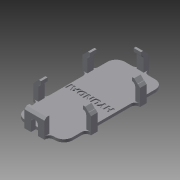
# Autodesk Inventor part: rev2
Saved by Autodesk Inventor 2015 SP2 (Build 190223200, 223)
## iProperties
Created: 2015-11-04
Part Number: rev2
Material: Generic
Document SubType Name: Modeling
Designer: KC-019
Density: 1 g/cm^3
Appearance: Default
Author: KC-019
Autodesk Inventor part; units mm, degrees
ref_plane "YZ Plane" through (0, 0, 0) normal (1, 0, 0) x (0, 1, 0)
ref_plane "XZ Plane" through (0, 0, 0) normal (0, 1, 0) x (-1, 0, 0)
ref_plane "XY Plane" through (0, 0, 0) normal (0, 0, 1) x (1, 0, 0)
sketch "Sketch1" plane through (0, 0, 0) normal (0, 0, 1) x (1, 0, 0)
  line L0 (0, 0) -> (44, 0)
  line L1 (44, 0) -> (44, 92)
  line L2 (44, 92) -> (0, 92)
  line L3 (0, 92) -> (0, 0)
  dimension "d0" = 44
  dimension "d1" = 92
  constraints: 8 end point, 2 parallel, 1 horizontal, 1 perpendicular
  measures "d0" distance of L2.end L1.end
  measures "d1" distance of L1.end L0.end
extrude "Extrusion1" add sketch "Sketch1" along normal blind 2.5
sketch "Sketch2" plane through (44, 0, 0) normal (1, 0, 0) x (0, 0, -1)
  line L0 (0, 0) -> (0, 92) projected
  line L1 (0, 46) -> (0, 23.5)
  line L2 (0, 92) -> (0, 0) projected
  line L3 (0, 46) -> (0, 68.5)
  line L4 (0, 68.5) -> (0, 65.5)
  line L5 (0, 65.5) -> (0, 71.5)
  line L6 (0, 65.5) -> (-17.1, 65.5)
  line L7 (-17.1, 65.5) -> (-17.1, 71.5)
  line L8 (-17.1, 71.5) -> (0, 71.5)
  line L9 (0, 71.5) -> (0, 65.5)
  line L10 (0, 46) -> (0, 49)
  line L11 (0, 23.5) -> (0, 20.5)
  line L12 (0, 20.5) -> (0, 26.5)
  line L13 (0, 20.5) -> (-17.1, 20.5)
  line L14 (-17.1, 20.5) -> (-17.1, 26.5)
  line L15 (-17.1, 26.5) -> (0, 26.5)
  line L16 (0, 26.5) -> (0, 20.5)
  dimension "d4" = 22.5
  dimension "d5" = 22.5
  dimension "d6" = 3
  dimension "d7" = 6
  dimension "d8" = 17.1
  dimension "d10" = 3
  dimension "d11" = 6
  dimension "d12" = 17.1
  constraints: 30 end point, 7 point on line, 4 parallel, 2 horizontal, 2 perpendicular, 1 midpoint
  measures "d4" distance of L1.start L1.end
  measures "d5" distance of L1.start L3.end
  measures "d6" distance of L3.end L4.end
  measures "d7" distance of L4.end L5.end
  measures "d8" distance of L7.end L8.end
  measures "d10" distance of L1.end L11.end
  measures "d11" distance of L11.end L12.end
  measures "d12" distance of L14.end L15.end
extrude "Extrusion2" add sketch "Sketch2" along normal blind 4.445
fillet "Fillet1" radius 4 4 edges at (44, 20.5, 1.25) (44, 65.5, 1.25) (44, 26.5, 1.25) (44, 71.5, 1.25)
chamfer "Chamfer1" distance 2 angle 45 2 edges at (48.445, 68.5, 17.1) (48.445, 23.5, 17.1)
sketch "Sketch3" plane through (0, 0, 0) normal (-1, 0, 0) x (0, 0, 1)
  line L0 (0, 92) -> (0, 0) projected
  line L1 (0, 46) -> (0, 26.5)
  line L2 (0, 46) -> (0, 65.5)
  line L3 (0, 26.5) -> (17.1, 26.5)
  line L4 (17.1, 26.5) -> (17.1, 20.5)
  line L5 (17.1, 20.5) -> (0, 20.5)
  line L6 (0, 20.5) -> (0, 26.5)
  line L7 (0, 65.5) -> (17.1, 65.5)
  line L8 (17.1, 65.5) -> (17.1, 71.5)
  line L9 (17.1, 71.5) -> (0, 71.5)
  line L10 (0, 71.5) -> (0, 65.5)
  constraints: 20 end point, 4 parallel, 2 horizontal, 2 perpendicular, 1 collinear, 1 midpoint, 1 vertical
extrude "Extrusion3" add sketch "Sketch3" along normal blind 4.445
chamfer "Chamfer2" distance 2 angle 45 2 edges at (-4.445, 68.5, 17.1) (-4.445, 23.5, 17.1)
fillet "Fillet2" radius 4 4 edges at (0, 65.5, 1.25) (0, 20.5, 1.25) (0, 71.5, 1.25) (0, 26.5, 1.25)
sketch "Sketch4" plane through (0, 92, 0) normal (0, 1, 0) x (1, 0, 0)
  line L0 (44, 0) -> (0, 0) projected
  line L1 (22, 0) -> (18.75, 0)
  line L2 (18.75, 0) -> (25.35, 0)
  line L3 (25.35, 0) -> (18.75, 0)
  line L4 (18.75, 0) -> (18.75, -17.1)
  line L5 (18.75, -17.1) -> (25.35, -17.1)
  line L6 (25.35, -17.1) -> (25.35, 0)
  dimension "d25" = 3.25
  dimension "d26" = 6.6
  dimension "d27" = 17.1
  constraints: 12 end point, 2 parallel, 2 point on line, 1 horizontal, 1 midpoint, 1 perpendicular
  measures "d25" distance of L1.start L1.end
  measures "d26" distance of L1.end L2.end
  measures "d27" distance of L4.end L3.end
extrude "Extrusion4" add sketch "Sketch4" along normal blind 4.445
fillet "Fillet3" radius 4 2 edges at (18.75, 92, 1.25) (25.35, 92, 1.25)
chamfer "Chamfer3" distance 2 angle 45 1 edges at (22.05, 96.445, 17.1)
sketch "Sketch5" plane through (0, 0, 0) normal (0, -1, 0) x (1, 0, 0)
  line L0 (25.35, 0) -> (18.75, 0) projected
  line L1 (22.05, 0) -> (24.59, 0)
  line L2 (24.59, 0) -> (18.24, 0)
  line L3 (24.59, 0) -> (30.59, 0)
  line L4 (30.59, 0) -> (30.59, 17.1)
  line L5 (30.59, 17.1) -> (24.59, 17.1)
  line L6 (24.59, 8.6399) -> (24.59, 0)
  line L7 (18.24, 0) -> (12.24, 0)
  line L8 (12.24, 0) -> (12.24, 17.1)
  line L9 (12.24, 17.1) -> (18.24, 17.1)
  line L10 (18.24, 8.6399) -> (18.24, 0)
  line L11 (24.59, 17.1) -> (18.24, 17.1)
  line L12 (21.59, 11.6399) -> (21.24, 11.6399)
  arc A0 (24.59, 8.6399) -> (21.59, 11.6399) centre (21.59, 8.6399) ccw
  arc A1 (21.24, 11.6399) -> (18.24, 8.6399) centre (21.24, 8.6399) ccw
  point P0 (0, 0)
  dimension "d34" = 2.54
  dimension "d35" = 6.35
  dimension "d36" = 6
  dimension "d37" = 17.1
  dimension "d38" = 6
  dimension "d39" = 3
  constraints: 24 end point, 5 point on line, 4 parallel, 4 point on circle, 4 tangent, 3 horizontal, 3 perpendicular, 2 centre point, 1 equal radius, 1 midpoint
  measures "d34" distance of L1.start L1.end
  measures "d35" distance of L1.end L2.end
  measures "d36" distance of L5.end L4.end
  measures "d37" distance of L4.end L3.end
  measures "d38" distance of L8.end L9.end
  measures "d39" radius of A0
extrude "Extrusion5" add sketch "Sketch5" along normal blind 4.445 contours L0 L6 A0 L12 A1 L10 L7 L8 L9 L11 L5 L4 L3
chamfer "Chamfer4" distance 2 angle 45 1 edges at (21.415, -4.445, 17.1)
fillet "Fillet4" radius 4 2 edges at (12.24, 0, 1.25) (30.59, 0, 1.25)
sketch "Sketch6" plane through (0, 0, 2.5) normal (0, 0, 1) x (1, 0, 0)
  line L0 (38.1695, 44.3728) -> (3.8106, 44.3728) construction
  line L1 (3.8106, 44.3728) -> (3.8106, 53.6459) construction
  line L2 (3.8106, 53.6459) -> (38.1695, 53.6459) construction
  line L3 (38.1695, 53.6459) -> (38.1695, 44.3728) construction
  line L4 (41.156, 49.8958) -> (40.9991, 47.6949)
  line L5 (40.9991, 47.6949) -> (40.9299, 46.0938)
  line L6 (40.9299, 46.0938) -> (40.9068, 45.3786)
  spline S0 degree 2 poles (40.9068, 45.3786) (40.9022, 45.0695) (40.9022, 44.7834) knots 0 0 0 1 1 1
  line L7 (40.9022, 44.7834) -> (40.9022, 44.3958)
  spline S1 degree 2 poles (40.9022, 44.3958) (40.2701, 44.4051) (39.9563, 44.4051) knots 0 0 0 1 1 1
  spline S2 degree 2 poles (39.9563, 44.4051) (39.7117, 44.4051) (39.1027, 44.3958) knots 0 0 0 1 1 1
  spline S3 degree 2 poles (39.1027, 44.3958) (39.1996, 45.554) (39.2273, 46.4399) knots 0 0 0 1 1 1
  line L8 (39.2273, 46.4399) -> (37.0402, 46.4399)
  spline S4 degree 2 poles (37.0402, 46.4399) (37.0217, 46.1077) (36.9848, 44.9818) (36.9848, 44.7742) knots 0 0 0 1 2 2 2
  spline S5 degree 2 poles (36.9848, 44.7742) (36.9848, 44.6681) (36.9894, 44.3958) knots 0 0 0 1 1 1
  line L9 (36.9894, 44.3958) -> (36.0343, 44.4051)
  spline S6 degree 2 poles (36.0343, 44.4051) (35.8821, 44.4051) (35.1853, 44.3958) knots 0 0 0 1 1 1
  spline S7 degree 2 poles (35.1853, 44.3958) (35.333, 46.4676) (35.416, 48.4839) (35.416, 49.8958) knots 0 0 0 1 2 2 2
  line L10 (35.416, 49.8958) -> (36.2927, 49.8866)
  spline S8 degree 2 poles (36.2927, 49.8866) (36.4911, 49.8866) (37.234, 49.8958) knots 0 0 0 1 1 1
  spline S9 degree 2 poles (37.234, 49.8958) (37.1325, 48.9361) (37.0956, 47.6626) knots 0 0 0 1 1 1
  line L11 (37.0956, 47.6626) -> (39.2919, 47.6626)
  line L12 (39.2919, 47.6626) -> (39.3611, 49.8958)
  line L13 (39.3611, 49.8958) -> (40.2931, 49.8866)
  spline S10 degree 2 poles (40.2931, 49.8866) (40.4731, 49.8866) (41.156, 49.8958) knots 0 0 0 1 1 1
  spline S11 degree 2 poles (33.2566, 49.8958) (33.2151, 49.5682) (33.1044, 48.0087) (33.1044, 47.6857) knots 0 0 0 1 2 2 2
  line L14 (33.1044, 47.6857) -> (34.9454, 44.3958)
  spline S12 degree 2 poles (34.9454, 44.3958) (34.3409, 44.4051) (33.9441, 44.4051) knots 0 0 0 1 1 1
  spline S13 degree 2 poles (33.9441, 44.4051) (33.5658, 44.4051) (33.0398, 44.3958) knots 0 0 0 1 1 1
  spline S14 degree 2 poles (33.0398, 44.3958) (32.8783, 44.8019) (32.3246, 45.9185) (32.1492, 46.3568) knots 0 0 0 1 2 2 2
  spline S15 degree 2 poles (32.1492, 46.3568) (31.6878, 45.5401) (31.1249, 44.6219) (31.0003, 44.3958) knots 0 0 0 1 2 2 2
  spline S16 degree 2 poles (31.0003, 44.3958) (30.4882, 44.4051) (30.0175, 44.4051) knots 0 0 0 1 1 1
  spline S17 degree 2 poles (30.0175, 44.4051) (29.7684, 44.4051) (29.1132, 44.3958) knots 0 0 0 1 1 1
  line L15 (29.1132, 44.3958) -> (30.885, 47.0074)
  spline S18 degree 2 poles (30.885, 47.0074) (31.411, 47.7872) (31.411, 47.8241) knots 0 0 0 1 1 1
  line L16 (31.411, 47.8241) -> (31.4156, 47.8656)
  line L17 (31.4156, 47.8656) -> (31.4156, 47.9025)
  line L18 (31.4156, 47.9025) -> (31.4202, 47.9441)
  line L19 (31.4202, 47.9441) -> (31.4479, 48.5577)
  spline S19 degree 2 poles (31.4479, 48.5577) (31.4756, 49.1622) (31.4894, 49.8958) knots 0 0 0 1 1 1
  spline S20 degree 2 poles (31.4894, 49.8958) (32.057, 49.8866) (32.3707, 49.8866) knots 0 0 0 1 1 1
  spline S21 degree 2 poles (32.3707, 49.8866) (32.6891, 49.8866) (33.2566, 49.8958) knots 0 0 0 1 1 1
  spline S22 degree 2 poles (28.864, 44.3958) (28.2365, 44.4051) (27.9781, 44.4051) knots 0 0 0 1 1 1
  spline S23 degree 2 poles (27.9781, 44.4051) (27.6551, 44.4051) (27.1199, 44.3958) knots 0 0 0 1 1 1
  line L20 (27.1199, 44.3958) -> (27.2399, 46.1077)
  spline S24 degree 2 poles (27.2399, 46.1077) (27.2768, 46.5921) (27.3137, 47.4365) (27.3137, 47.598) knots 0 0 0 1 2 2 2
  spline S25 degree 2 poles (27.3137, 47.598) (27.3137, 47.9072) (27.226, 48.3178) (26.9907, 48.6039) (26.5754, 48.7469) (26.3493, 48.7469) knots 0 0 0 1 2 3 4 4 4
  spline S26 degree 2 poles (26.3493, 48.7469) (26.1555, 48.7469) (25.9848, 48.6962) knots 0 0 0 1 1 1
  spline S27 degree 2 poles (25.9848, 48.6962) (25.851, 48.65) (25.7449, 48.5762) knots 0 0 0 1 1 1
  spline S28 degree 2 poles (25.7449, 48.5762) (25.6526, 48.5024) (25.5834, 48.4055) knots 0 0 0 1 1 1
  spline S29 degree 2 poles (25.5834, 48.4055) (25.5003, 48.2901) (25.4357, 48.1194) knots 0 0 0 1 1 1
  spline S30 degree 2 poles (25.4357, 48.1194) (25.3711, 47.9533) (25.3388, 47.6949) knots 0 0 0 1 1 1
  spline S31 degree 2 poles (25.3388, 47.6949) (25.3019, 47.4319) (25.2419, 46.4952) knots 0 0 0 1 1 1
  spline S32 degree 2 poles (25.2419, 46.4952) (25.1912, 45.7016) (25.1635, 45.0372) knots 0 0 0 1 1 1
  spline S33 degree 2 poles (25.1635, 45.0372) (25.1358, 44.3958) (25.1174, 44.3958) knots 0 0 0 1 1 1
  spline S34 degree 2 poles (25.1174, 44.3958) (24.5083, 44.3958) (24.1576, 44.3958) knots 0 0 0 1 1 1
  line L21 (24.1576, 44.3958) -> (23.3409, 44.3958)
  line L22 (23.3409, 44.3958) -> (23.5393, 47.2566)
  spline S35 degree 2 poles (23.5393, 47.2566) (23.544, 47.3396) (23.544, 47.3904) knots 0 0 0 1 1 1
  spline S36 degree 2 poles (23.544, 47.3904) (23.5578, 48.2301) (23.7331, 48.9176) (24.1346, 49.4252) (24.9097, 49.8312) (25.8925, 50.002) (26.3955, 50.002) knots 0 0 0 1 2 3 4 5 5 5
  spline S37 degree 2 poles (26.3955, 50.002) (26.8477, 50.002) (27.2675, 49.9374) knots 0 0 0 1 1 1
  spline S38 degree 2 poles (27.2675, 49.9374) (27.6551, 49.8728) (28.2734, 49.6282) (28.5041, 49.4621) knots 0 0 0 1 2 2 2
  spline S39 degree 2 poles (28.5041, 49.4621) (28.7117, 49.3098) (28.9378, 48.9915) (29.0024, 48.77) knots 0 0 0 1 2 2 2
  spline S40 degree 2 poles (29.0024, 48.77) (29.0763, 48.5208) (29.0763, 48.2348) knots 0 0 0 1 1 1
  spline S41 degree 2 poles (29.0763, 48.2348) (29.0763, 48.1379) (29.0578, 47.7457) (29.0301, 47.3765) knots 0 0 0 1 2 2 2
  line L23 (29.0301, 47.3765) -> (28.9794, 46.7352)
  spline S42 degree 2 poles (28.9794, 46.7352) (28.9609, 46.4814) (28.9332, 45.9877) knots 0 0 0 1 1 1
  line L24 (28.9332, 45.9877) -> (28.864, 44.3958)
  line L25 (22.6857, 49.8958) -> (22.6073, 49.0515)
  line L26 (22.6073, 49.0515) -> (22.4504, 46.1815)
  line L27 (22.4504, 46.1815) -> (22.4043, 45.0233)
  line L28 (22.4043, 45.0233) -> (22.4043, 44.3958)
  spline S43 degree 2 poles (22.4043, 44.3958) (21.7814, 44.4051) (21.3015, 44.4051) knots 0 0 0 1 1 1
  spline S44 degree 2 poles (21.3015, 44.4051) (20.9601, 44.4051) (20.3372, 44.3958) knots 0 0 0 1 1 1
  line L29 (20.3372, 44.3958) -> (18.6115, 47.5242)
  line L30 (18.6115, 47.5242) -> (18.3716, 47.9856)
  spline S45 degree 2 poles (18.3716, 47.9856) (18.33, 47.3073) (18.2378, 44.8619) (18.2378, 44.3958) knots 0 0 0 1 2 2 2
  spline S46 degree 2 poles (18.2378, 44.3958) (17.744, 44.4051) (17.4441, 44.4051) knots 0 0 0 1 1 1
  spline S47 degree 2 poles (17.4441, 44.4051) (17.3103, 44.4051) (16.6551, 44.3958) knots 0 0 0 1 1 1
  line L31 (16.6551, 44.3958) -> (16.752, 45.5955)
  line L32 (16.752, 45.5955) -> (16.932, 48.9315)
  line L33 (16.932, 48.9315) -> (16.955, 49.8958)
  spline S48 degree 2 poles (16.955, 49.8958) (17.481, 49.8866) (17.9332, 49.8866) knots 0 0 0 1 1 1
  spline S49 degree 2 poles (17.9332, 49.8866) (18.3162, 49.8866) (18.9852, 49.8958) knots 0 0 0 1 1 1
  spline S50 degree 2 poles (18.9852, 49.8958) (19.1929, 49.499) (19.2944, 49.3237) knots 0 0 0 1 1 1
  line L34 (19.2944, 49.3237) -> (19.9727, 48.1748)
  spline S51 degree 2 poles (19.9727, 48.1748) (20.3049, 47.6119) (20.5909, 47.0951) knots 0 0 0 1 1 1
  spline S52 degree 2 poles (20.5909, 47.0951) (20.7755, 46.7675) (20.9739, 46.3753) knots 0 0 0 1 1 1
  line L35 (20.9739, 46.3753) -> (21.057, 48.2855)
  line L36 (21.057, 48.2855) -> (21.0985, 49.8958)
  spline S53 degree 2 poles (21.0985, 49.8958) (21.5968, 49.8866) (21.8552, 49.8866) knots 0 0 0 1 1 1
  spline S54 degree 2 poles (21.8552, 49.8866) (22.0767, 49.8866) (22.6857, 49.8958) knots 0 0 0 1 1 1
  spline S55 degree 2 poles (15.9076, 49.8958) (15.82, 48.9776) (15.7877, 48.4239) knots 0 0 0 1 1 1
  spline S56 degree 2 poles (15.7877, 48.4239) (15.7369, 47.6026) (15.6908, 46.2968) knots 0 0 0 1 1 1
  spline S57 degree 2 poles (15.6908, 46.2968) (15.6539, 45.3002) (15.6539, 44.8665) knots 0 0 0 1 1 1
  line L37 (15.6539, 44.8665) -> (15.6539, 44.3958)
  spline S58 degree 2 poles (15.6539, 44.3958) (15.1832, 44.4097) (14.8418, 44.4097) knots 0 0 0 1 1 1
  spline S59 degree 2 poles (14.8418, 44.4097) (14.5096, 44.4097) (13.4391, 44.3728) (12.9685, 44.3728) knots 0 0 0 1 2 2 2
  spline S60 degree 2 poles (12.9685, 44.3728) (12.4286, 44.3728) (11.6119, 44.502) (10.906, 44.9034) (10.4307, 45.554) (10.1815, 46.4306) (10.1815, 46.8921) knots 0 0 0 1 2 3 4 5 5 5
  spline S61 degree 2 poles (10.1815, 46.8921) (10.1815, 47.3489) (10.3753, 48.1932) (10.7214, 48.8669) (11.1828, 49.356) (11.4827, 49.5313) knots 0 0 0 1 2 3 4 4 4
  spline S62 degree 2 poles (11.4827, 49.5313) (11.7042, 49.6559) (12.1564, 49.8035) (12.5486, 49.8497) knots 0 0 0 1 2 2 2
  spline S63 degree 2 poles (12.5486, 49.8497) (12.9823, 49.8958) (13.536, 49.8958) knots 0 0 0 1 1 1
  line L38 (13.536, 49.8958) -> (15.1602, 49.882)
  spline S64 degree 2 poles (15.1602, 49.882) (15.3909, 49.882) (15.9076, 49.8958) knots 0 0 0 1 1 1
  spline S65 degree 2 poles (14.1635, 48.6823) (13.942, 48.7008) (13.7021, 48.7008) knots 0 0 0 1 1 1
  spline S66 degree 2 poles (13.7021, 48.7008) (13.2914, 48.7008) (12.6455, 48.5577) (12.161, 48.0825) (11.9257, 47.335) (11.9257, 46.9474) knots 0 0 0 1 2 3 4 4 4
  spline S67 degree 2 poles (11.9257, 46.9474) (11.9257, 46.4676) (12.2717, 45.8124) (12.8485, 45.554) (13.3422, 45.554) knots 0 0 0 1 2 3 3 3
  spline S68 degree 2 poles (13.3422, 45.554) (13.6329, 45.554) (14.0297, 45.577) knots 0 0 0 1 1 1
  line L39 (14.0297, 45.577) -> (14.1635, 48.6823)
  line L40 (10.2554, 49.8958) -> (9.9232, 49.3145)
  line L41 (9.9232, 49.3145) -> (7.8376, 45.3925)
  line L42 (7.8376, 45.3925) -> (7.6161, 44.9541)
  spline S69 degree 2 poles (7.6161, 44.9541) (7.5192, 44.7603) (7.3485, 44.3958) knots 0 0 0 1 1 1
  spline S70 degree 2 poles (7.3485, 44.3958) (6.6379, 44.4051) (6.3103, 44.4051) knots 0 0 0 1 1 1
  spline S71 degree 2 poles (6.3103, 44.4051) (5.7428, 44.4051) (5.2583, 44.3958) knots 0 0 0 1 1 1
  line L43 (5.2583, 44.3958) -> (4.6723, 46.0754)
  line L44 (4.6723, 46.0754) -> (3.4773, 49.3052)
  line L45 (3.4773, 49.3052) -> (3.2419, 49.8958)
  spline S72 degree 2 poles (3.2419, 49.8958) (3.9387, 49.8866) (4.0863, 49.8866) knots 0 0 0 1 1 1
  spline S73 degree 2 poles (4.0863, 49.8866) (4.4278, 49.8866) (5.083, 49.8958) knots 0 0 0 1 1 1
  spline S74 degree 2 poles (5.083, 49.8958) (5.2583, 49.2314) (5.5951, 48.3317) knots 0 0 0 1 1 1
  line L46 (5.5951, 48.3317) -> (7.6253, 48.3317)
  spline S75 degree 2 poles (7.6253, 48.3317) (7.9714, 49.0422) (8.3498, 49.8958) knots 0 0 0 1 1 1
  spline S76 degree 2 poles (8.3498, 49.8958) (9.0972, 49.8866) (9.268, 49.8866) knots 0 0 0 1 1 1
  spline S77 degree 2 poles (9.268, 49.8866) (9.5725, 49.8866) (10.2554, 49.8958) knots 0 0 0 1 1 1
  line L47 (7.1362, 47.1597) -> (5.8858, 47.1597)
  spline S78 degree 2 poles (5.8858, 47.1597) (6.3518, 45.7385) (6.3934, 45.5955) knots 0 0 0 1 1 1
  spline S79 degree 2 poles (6.3934, 45.5955) (6.661, 46.1861) (6.8456, 46.5645) knots 0 0 0 1 1 1
  line L48 (6.8456, 46.5645) -> (7.1362, 47.1597)
  spline S80 degree 2 poles (2.8036, 49.8958) (2.5683, 46.6614) (2.5683, 44.9172) knots 0 0 0 1 1 1
  line L49 (2.5683, 44.9172) -> (2.5729, 44.3958)
  spline S81 degree 2 poles (2.5729, 44.3958) (1.8669, 44.4051) (1.6316, 44.4051) knots 0 0 0 1 1 1
  spline S82 degree 2 poles (1.6316, 44.4051) (1.5209, 44.4051) (0.7642, 44.3958) knots 0 0 0 1 1 1
  spline S83 degree 2 poles (0.7642, 44.3958) (0.838, 45.3002) (0.8841, 46.1123) knots 0 0 0 1 1 1
  spline S84 degree 2 poles (0.8841, 46.1123) (0.9395, 47.2427) (0.9903, 49.2037) (0.9903, 49.8958) knots 0 0 0 1 2 2 2
  line L50 (0.9903, 49.8958) -> (1.8116, 49.8866)
  spline S85 degree 2 poles (1.8116, 49.8866) (2.0561, 49.8866) (2.8036, 49.8958) knots 0 0 0 1 1 1
  point P0 (0, 0)
  constraints: 2 other
extrude "Extrusion6" cut sketch "Sketch6" against normal blind 1
sketch "Sketch7" plane through (44, 20.5, 17.1) normal (0, 0, 1) x (1, 0, 0)
  line L0 (0, 0) -> (4, 0) projected
  line L1 (2, 0) -> (-3, 0)
  line L2 (-3, 0) -> (-3, 6)
  line L3 (-3, 6) -> (2, 6)
  line L4 (2, 6) -> (2, 0)
  line L5 (2, 51) -> (-3, 51)
  line L6 (-3, 51) -> (-3, 45)
  line L7 (-3, 45) -> (2, 45)
  line L8 (2, 45) -> (2, 51)
  line L9 (-46.445, 51) -> (-41.445, 51)
  line L10 (-41.445, 51) -> (-41.445, 45)
  line L11 (-41.445, 45) -> (-46.445, 45)
  line L12 (-46.445, 45) -> (-46.445, 51)
  line L13 (-46.445, 6) -> (-41.445, 6)
  line L14 (-41.445, 6) -> (-41.445, 0)
  line L15 (-41.445, 0) -> (-46.445, 0)
  line L16 (-46.445, 0) -> (-46.445, 6)
  line L17 (-18.65, 73.945) -> (-25.25, 73.945)
  line L18 (-25.25, 73.945) -> (-25.25, 68.9641)
  line L19 (-25.25, 68.9641) -> (-18.65, 68.9641)
  line L20 (-18.65, 68.9641) -> (-18.65, 73.945)
  point P0 (-44, -20.5)
  dimension "d48" = 5
  dimension "d49" = 5
  constraints: 40 end point, 10 parallel, 5 horizontal, 5 perpendicular, 1 midpoint, 1 point on line
  measures "d48" distance of L2.end L3.end
  measures "d49" distance of L10.end L11.end
extrude "Extrusion7" add sketch "Sketch7" along normal blind 3
fillet "Fillet5" radius 3 5 edges at (44, 68.5, 17.1) (44, 23.5, 17.1) (0, 68.5, 17.1) (0, 23.5, 17.1) (22.05, 92, 17.1)
chamfer "Chamfer5" distance 3 angle 45 5 edges at (-2.445, 23.5, 20.1) (-2.445, 68.5, 20.1) (46, 23.5, 20.1) (46, 68.5, 20.1) (22.05, 94.445, 20.1)
fillet "Fillet6" radius 8 4 edges at (0, 0, 1.25) (44, 0, 1.25) (44, 92, 1.25) (0, 92, 1.25)
body "Solid1"
